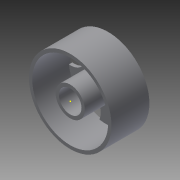
# Autodesk Inventor part: WheelDE
Saved by Autodesk Inventor 2015 (Build 190159000, 159)
## iProperties
Created: 2017-12-01
Part Number: WheelDE
Material: Generic
Document SubType Name: Modeling
Designer: Administrator
Density: 1 g/cm^3
Appearance: Default
Author: Administrator
Autodesk Inventor part; units mm, degrees
ref_plane "YZ Plane" through (0, 0, 0) normal (1, 0, 0) x (0, 1, 0)
ref_plane "XZ Plane" through (0, 0, 0) normal (0, 1, 0) x (-1, 0, 0)
ref_plane "XY Plane" through (0, 0, 0) normal (0, 0, 1) x (1, 0, 0)
sketch "Sketch1" plane through (0, 0, 0) normal (0, 0, 1) x (1, 0, 0)
  circle A0 centre (0, 0) radius 5.588
  circle A1 centre (0, 0) radius 4.318
  circle A2 centre (0, 0) radius 14.478
  circle A3 centre (0, 0) radius 15.748
  dimension "d0" = 1.27
  dimension "d1" = 11.176
  dimension "d2" = 1.27
  dimension "d3" = 8.89
  constraints: 4 centre point, 4 coincident
  measures "d0" radial gap between concentric circles of A1 A0
  measures "d1" diameter of A0
  measures "d2" radial gap between concentric circles of A2 A3
  measures "d3" radial gap between concentric circles of A2 A0
extrude "Extrusion1" add sketch "Sketch1" along normal blind 14.478
sketch "Sketch3" plane through (0, 0, 14.478) normal (0, 0, 1) x (1, 0, 0)
  point P0 (0, 0)
extrude "Extrusion2" add sketch "Sketch1" along normal mid plane 1.27 contours A0 | A2
sketch "Sketch4" plane through (0, 0, -0.635) normal (0, 0, -1) x (-1, 0, 0)
  arc A0 (-6.1954, 13.0855) -> (6.1954, 13.0855) centre (0, 14.478) ccw
  arc A1 (6.1954, 13.0855) -> (-6.1954, 13.0855) centre (0, 0) ccw
  arc A2 (-14.3595, -1.8486) -> (-10.5305, 9.9358) centre (-13.7694, 4.4739) ccw
  arc A3 (-10.5305, 9.9358) -> (-14.3595, -1.8486) centre (0, 0) ccw
  arc A4 (-2.6792, -14.2279) -> (-12.7036, -6.9448) centre (-8.51, -11.7129) ccw
  arc A5 (-12.7036, -6.9448) -> (-2.6792, -14.2279) centre (0, 0) ccw
  arc A6 (12.7036, -6.9448) -> (2.6792, -14.2279) centre (8.51, -11.7129) ccw
  arc A7 (2.6792, -14.2279) -> (12.7036, -6.9448) centre (0, 0) ccw
  arc A8 (10.5305, 9.9358) -> (14.3595, -1.8486) centre (13.7694, 4.4739) ccw
  arc A9 (14.3595, -1.8486) -> (10.5305, 9.9358) centre (0, 0) ccw
  point P0 (0, 0)
  dimension "d8" = 12.7
  dimension "d11" = 360
  constraints: 25 point on circle, 10 centre point, 31 other
  measures "d8" diameter of A0
extrude "Extrusion3" cut sketch "Sketch4" against normal blind 2.54
body "Solid1"
